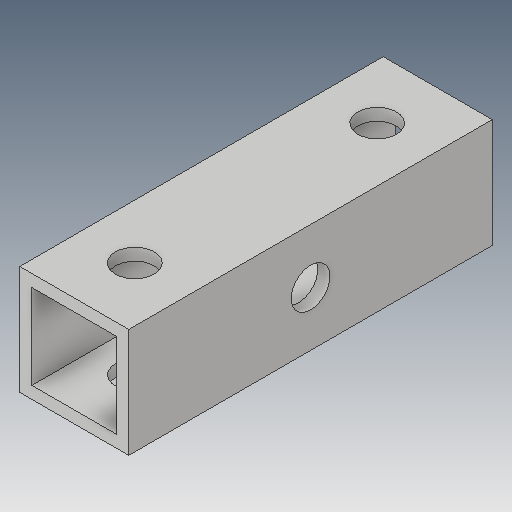
# Autodesk Inventor part: SqPipeminin
Saved by Autodesk Inventor 2019.4 (Build 234330000, 330)
## iProperties
Created: 2019-06-12
Part Number: SqPipeminin
Material: Generic
Document SubType Name: Modeling
Designer: AzLIer
Density: 1 g/cm^3
Appearance: Default
Mass: 0.911745 g
Surface Area: 19.4781 cm^2
Volume: 0.911745 cm^3
Author: AzLIer
Autodesk Inventor part; units mm, degrees
ref_plane "YZ Plane" through (0, 0, 0) normal (1, 0, 0) x (0, 1, 0)
ref_plane "XZ Plane" through (0, 0, 0) normal (0, 1, 0) x (-1, 0, 0)
ref_plane "XY Plane" through (0, 0, 0) normal (0, 0, 1) x (1, 0, 0)
sketch "スケッチ1" plane through (0, 0, 0) normal (0, 0, 1) x (1, 0, 0)
  line L0 (4.5, -4.5) -> (-4.5, -4.5)
  line L1 (-4.5, -4.5) -> (-4.5, 4.5)
  line L2 (-4.5, 4.5) -> (4.5, 4.5)
  line L3 (4.5, 4.5) -> (4.5, -4.5)
  line L4 (4.5, -4.5) -> (-4.5, 4.5) construction
  line L5 (-4.5, -4.5) -> (4.5, 4.5) construction
  point P0 (0, 0)
  dimension "d0" = 9
  dimension "d1" = 9
  constraints: 12 end point, 2 midpoint, 2 parallel, 1 horizontal, 1 perpendicular
  measures "d0" distance of L1.end L2.end
  measures "d1" distance of L0.end L1.end
extrude "押し出し1" add sketch "スケッチ1" along normal blind 30
shell "シェル1" thickness 1 removed faces 2 at (1.5, -1.5, 0) at (1.5, -1.5, 30)
sketch "スケッチ2" plane through (-4.5, 4.5, 0) normal (0, 1, 0) x (1, 0, 0)
  line L0 (0, 0) -> (9, 0) projected
  point P0 (4.5, 0)
  point P1 (4.5, -5)
  point P2 (4.5, -25)
  point P3 (4.5, 0)
  dimension "d5" = 20
  dimension "d6" = 5
  constraints: 2 vertical alignment, 1 midpoint
  measures "d5" distance of point (4.5, -25) point (4.5, -5)
  measures "d6" distance from line of L0 point (4.5, -5)
hole "穴1" at (0, 4.5, 5) at (0, 4.5, 25) direction (0, -1, 0) diameter 3.2 end through all
sketch "スケッチ3" plane through (4.5, -4.5, 0) normal (1, 0, 0) x (0, 0, -1)
  line L0 (0, 9) -> (0, 0) projected
  line L1 (0, 9) -> (-30, 9) projected
  line L2 (-30, 0) -> (-30, 9) projected
  line L3 (0, 0) -> (-30, 0) projected
  point P0 (0, 4.5)
  point P1 (-15, 4.5)
  point P2 (-15, 9)
  point P3 (0, 4.5)
  constraints: 2 midpoint, 1 horizontal alignment, 1 vertical alignment
hole "穴2" at (4.5, 0, 15) direction (-1, 0, 0) diameter 3.2 end through all
